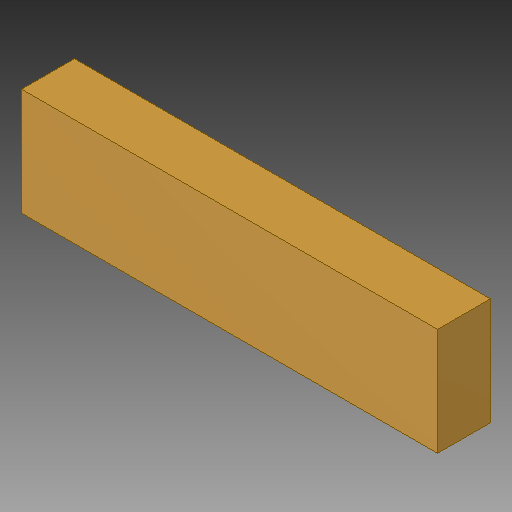
# Autodesk Inventor part: 1N4148DO35-7
Saved by Autodesk Inventor 2017 (Build 210142000, 142)
## iProperties
Created: 2019-06-13
Part Number: 1N4148DO35-7
Material: Generic
Document SubType Name: Modeling
Designer: Marc
Density: 1 g/cm^3
Appearance: DO35-7, 1N4148DO35-7
Author: Marc
Autodesk Inventor part; units mm, degrees
ref_plane "YZ Plane" through (0, 0, 0) normal (1, 0, 0) x (0, 1, 0)
ref_plane "XZ Plane" through (0, 0, 0) normal (0, 1, 0) x (-1, 0, 0)
ref_plane "XY Plane" through (0, 0, 0) normal (0, 0, 1) x (1, 0, 0)
sketch "DO35-7, 1N4148DO35-7_42" plane through (0, 0, 0) normal (0, 0, 1) x (1, 0, 0)
  line L0 (-3.81, 1.016) -> (4.064, 1.016)
  line L1 (4.064, 1.016) -> (4.064, -1.016)
  line L2 (4.064, -1.016) -> (-3.81, -1.016)
  line L3 (-3.81, -1.016) -> (-3.81, 1.016)
  constraints: 8 end point
extrude "Extrusion1" add sketch "DO35-7, 1N4148DO35-7_42" along normal blind 1
body "Solid1"
